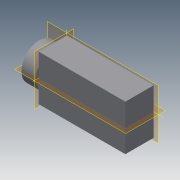
# Autodesk Inventor part: ST-PJ-312
Saved by Autodesk Inventor 2015 SP1 (Build 190203100, 203)
## iProperties
Created: 2016-01-28
Part Number: ST-PJ-312
Material: Generic
Document SubType Name: Modeling
Designer: Yamaura
Density: 1 g/cm^3
Appearance: Default
Author: Yamaura
Autodesk Inventor part; units mm, degrees
sketch "スケッチ1" plane through (0, 0, 0) normal (0, 1, 0) x (-1, 0, 0)
  point P0 (0, 0)
sketch "スケッチ2" plane through (0, 0, 0) normal (0, 0, 1) x (1, 0, 0)
  circle A0 centre (10.5, 0) radius 0.6
  line L0 (-2.22, 0) -> (13.32, 0) projected
  point P0 (0, 0)
  point P1 (0, 0)
  dimension "d0" = 1.2
  dimension "d3" = 10.5
  constraints: 1 centre point, 1 coincident, 1 horizontal alignment, 1 point on line
  measures "d0" diameter of A0
  measures "d3" distance of point (0, 0) point (10.5, 0)
extrude "押し出し1" add sketch "スケッチ2" against normal blind 0.5
sketch "スケッチ4" plane through (0, 0, 0) normal (0, 0, 1) x (1, 0, 0)
  line L0 (12, 3.15) -> (0, 3.15)
  line L1 (0, 3.15) -> (0, -3.15)
  line L2 (0, -3.15) -> (12, -3.15)
  line L3 (12, -3.15) -> (12, 3.15)
  point P0 (0, 0)
  dimension "d4" = 3.15
  dimension "d5" = 6.3
  dimension "d6" = 12
  constraints: 8 end point, 2 parallel, 1 horizontal, 1 midpoint, 1 perpendicular
  measures "d4" distance from line of L0 point (0, 0)
  measures "d5" distance of L2.end L0.start
  measures "d6" distance from line of L3 point (0, 0)
extrude "押し出し2" add sketch "スケッチ4" along normal blind 3.9
sketch "スケッチ5" plane through (0, 0, 0) normal (1, 0, 0) x (0, 1, 0)
  circle A0 centre (0, 1.8) radius 2.5
  point P0 (0, 0)
  dimension "d9" = 5
  dimension "d10" = 1.8
  constraints: 1 centre point
  measures "d9" diameter of A0
  measures "d10" distance of A0.centre point (0, 0)
extrude "押し出し3" add sketch "スケッチ5" against normal blind 2
sketch "スケッチ6" plane through (0, 0, 0) normal (0, 0, 1) x (1, 0, 0)
  line L0 (0, -1.5) -> (1.0909, -1.5)
  line L1 (1.0909, -1.5) -> (1.0909, 1.5)
  line L2 (1.0909, 1.5) -> (0, 1.5)
  line L3 (0, 1.5) -> (0, -1.5)
  line L4 (-4.8, 0) -> (14.8, 0) projected
  point P0 (0, 0)
  dimension "d13" = 3
  dimension "d14" = 1.5
  constraints: 8 end point, 2 parallel, 1 horizontal, 1 perpendicular
  measures "d13" distance of L0.end L1.end
  measures "d14" distance between parallel lines of L0 L4
extrude "押し出し4" add sketch "スケッチ6" against normal blind 0.5
